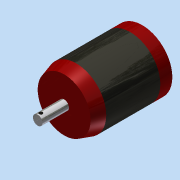
# Autodesk Inventor part: Motor
Saved by Autodesk Inventor 2015 (Build 190159000, 159)
## iProperties
Created: 2015-11-06
Part Number: Motor
Material: Aluminum 6061
Document SubType Name: Modeling
Designer: Raphael
Density: 2.7 g/cm^3
Appearance: Gunmetal
Mass: 341.324 g
Surface Area: 142.76 cm^2
Volume: 126.416 cm^3
Author: Raphael
Autodesk Inventor part; units mm, degrees
ref_plane "YZ Plane" through (0, 0, 0) normal (1, 0, 0) x (0, 1, 0)
sketch "Sketch2" plane through (0, 0, 0) normal (0, 0, 1) x (1, 0, 0)
  circle A0 centre (0, 0) radius 25
  dimension "d0" = 50
  constraints: 1 centre point, 1 coincident
  measures "d0" diameter of A0
extrude "Extrusion1" add sketch "Sketch2" along normal blind 65
sketch "Sketch3" plane through (0, 0, 65) normal (0, 0, 1) x (1, 0, 0)
  circle A0 centre (0, 0) radius 4
  dimension "d3" = 8
  constraints: 1 centre point, 1 coincident
  measures "d3" diameter of A0
extrude "Extrusion2" add sketch "Sketch3" along normal blind 22
ref_plane "Work Plane1" through (0, 0, 55) normal (0, 0, 1) x (1, 0, 0)
ref_plane "Work Plane2" through (0, 0, 10) normal (0, 0, -1) x (-1, 0, 0)
split_face "Split1"
split_face "Split2"
chamfer "Chamfer1" distance 3 distance2 10 1 edges at (-25, 0, 65) measured on face at (17.7191, -2.3134, 65)
sketch "Sketch4" plane through (0, 0, 0) normal (0, 1, 0) x (-1, 0, 0)
  line L0 (4, 87) -> (-4, 87) projected
  line L1 (-4, 65) -> (4, 65) projected
  circle A0 centre (0, 84.5) radius 1.5
  point P0 (0, 0)
  dimension "d11" = 3
  dimension "d12" = 2.5
  constraints: 1 centre point
  measures "d11" diameter of A0
  measures "d12" distance from line of A0.centre L0
extrude "Extrusion3" cut sketch "Sketch4" along normal through all both and the other way through all
body "Solid1"
